Autodesk Fusion 360 part; units mm, degrees
(part 2 of 2)
  spline S41 degree 3 poles (-24.3468, 0.9983) (-24.5744, 0.8236) (-24.8811, 0.6674) (-25.4193, 0.5131) (-25.7453, 0.4822) (-26.274, 0.5385) (-26.5708, 0.63) (-27.014, 0.8762) (-27.2402, 1.07) (-27.3913, 1.2669) (-27.4167, 1.3) (-27.4417, 1.3349) (-27.466, 1.3714) knots -0.320047 -0.320047 -0.320047 -0.320047 -0.233978 -0.233978 -0.152103 -0.152103 -0.074471 -0.074471 0 0 0 0.012509 0.012509 0.012509 0.012509
  spline S42 degree 3 poles (-32.2928, 13.0243) (-32.3014, 13.0672) (-32.3084, 13.1096) (-32.3138, 13.1509) (-32.3462, 13.397) (-32.3233, 13.694) (-32.184, 14.1815) (-32.0388, 14.456) (-31.7048, 14.8697) (-31.4524, 15.0784) (-30.9628, 15.3498) (-30.6354, 15.4563) (-30.351, 15.4937) knots -0.012509 -0.012509 -0.012509 -0.012509 0 0 0 0.074471 0.074471 0.152103 0.152103 0.233978 0.233978 0.320047 0.320047 0.320047 0.320047
  arc A22 (-32.2928, 13.0243) -> (-31.2194, 9.0185) centre (-0.3, 19.45) ccw
  spline S43 degree 3 poles (-28.303, 7.8508) (-28.5681, 7.741) (-28.9049, 7.6694) (-29.4646, 7.6597) (-29.7875, 7.7143) (-30.2836, 7.9055) (-30.5466, 8.0706) (-30.911, 8.4231) (-31.0793, 8.6689) (-31.1743, 8.8983) (-31.1903, 8.9368) (-31.2054, 8.977) (-31.2194, 9.0185) knots -0.320047 -0.320047 -0.320047 -0.320047 -0.233978 -0.233978 -0.152103 -0.152103 -0.074471 -0.074471 0 0 0 0.012509 0.012509 0.012509 0.012509
  spline S44 degree 3 poles (-32.8657, 21.5236) (-32.863, 21.5672) (-32.8587, 21.61) (-32.8533, 21.6513) (-32.8209, 21.8975) (-32.7219, 22.1784) (-32.4612, 22.6132) (-32.2499, 22.8408) (-31.8202, 23.1539) (-31.5224, 23.2902) (-30.9792, 23.4257) (-30.6354, 23.4437) (-30.351, 23.4063) knots -0.012509 -0.012509 -0.012509 -0.012509 0 0 0 0.074471 0.074471 0.152103 0.152103 0.233978 0.233978 0.320047 0.320047 0.320047 0.320047
  arc A23 (-32.8657, 21.5236) -> (-32.8657, 17.3764) centre (-0.3, 19.45) ccw
  spline S45 degree 3 poles (-30.351, 15.4937) (-30.6354, 15.4563) (-30.9792, 15.4743) (-31.5224, 15.6098) (-31.8202, 15.7461) (-32.2499, 16.0592) (-32.4612, 16.2868) (-32.7219, 16.7216) (-32.8209, 17.0025) (-32.8533, 17.2487) (-32.8587, 17.29) (-32.863, 17.3328) (-32.8657, 17.3764) knots -0.320047 -0.320047 -0.320047 -0.320047 -0.233978 -0.233978 -0.152103 -0.152103 -0.074471 -0.074471 0 0 0 0.012509 0.012509 0.012509 0.012509
  spline S46 degree 3 poles (-31.2194, 29.8815) (-31.2054, 29.923) (-31.1903, 29.9632) (-31.1743, 30.0017) (-31.0793, 30.2311) (-30.911, 30.4769) (-30.5466, 30.8294) (-30.2836, 30.9945) (-29.7875, 31.1857) (-29.4646, 31.2403) (-28.9049, 31.2306) (-28.5681, 31.159) (-28.303, 31.0492) knots -0.012509 -0.012509 -0.012509 -0.012509 0 0 0 0.074471 0.074471 0.152103 0.152103 0.233978 0.233978 0.320047 0.320047 0.320047 0.320047
  arc A24 (-31.2194, 29.8815) -> (-32.2928, 25.8757) centre (-0.3, 19.45) ccw
  spline S47 degree 3 poles (-30.351, 23.4063) (-30.6354, 23.4437) (-30.9628, 23.5502) (-31.4524, 23.8216) (-31.7048, 24.0303) (-32.0388, 24.444) (-32.184, 24.7185) (-32.3233, 25.206) (-32.3462, 25.503) (-32.3138, 25.7491) (-32.3084, 25.7904) (-32.3014, 25.8328) (-32.2928, 25.8757) knots -0.320047 -0.320047 -0.320047 -0.320047 -0.233978 -0.233978 -0.152103 -0.152103 -0.074471 -0.074471 0 0 0 0.012509 0.012509 0.012509 0.012509
  line L0 (-22.8918, 33) -> (-17.5918, 33)
  line L1 (-17.5918, 33) -> (-17.5918, 9.5)
  line L2 (-17.5918, 9.5) -> (-22.8918, 9.5)
  line L3 (-22.8918, 9.5) -> (-22.8918, 33)
  circle A25 centre (-0.3, 19.45) radius 4.05
  point P0 (-0.3, 19.45)
  dimension "d1967" = 2.1
  dimension "d2049" = 3
  constraint coincident P0 A0.centre
  measures "d1967" diameter of A0
extrude "Extrude11" add sketch "top_mount" against normal blind 5 contours A25 bodies 5 in component "Cover"
extrude "Extrude6'" cut sketch "top_mount" against normal through all contours A0 bodies 5 in component "Cover"
sketch "Sketch12" plane through (-21.6568, 0, 0) normal (1, 0, 0) x (0, 1, 0) in component "Cover"
  line L0 (-0.1526, -8.2) -> (-0.1526, 19.5)
  line L1 (-2.7, -8.2) -> (-0.1526, -8.2)
  line L2 (-36.2, -8.2) -> (-36.2, 6.4)
  spline S0 degree 3 poles (-19.45, -5.6) (-19.3181, -5.6) (-19.1775, -5.5736) (-18.9188, -5.4665) (-18.8008, -5.3857) (-18.6143, -5.1992) (-18.5335, -5.0812) (-18.4264, -4.8225) (-18.4, -4.6819) (-18.4, -4.4181) (-18.4264, -4.2775) (-18.5335, -4.0188) (-18.6143, -3.9008) (-18.8008, -3.7143) (-18.9188, -3.6335) (-19.1775, -3.5264) (-19.3181, -3.5) (-19.45, -3.5) knots 0.158223 0.158223 0.158223 0.158223 0.197779 0.197779 0.237335 0.237335 0.276891 0.276891 0.316447 0.316447 0.356002 0.356002 0.395558 0.395558 0.435114 0.435114 0.47467 0.47467 0.47467 0.47467 construction
  spline S1 degree 3 poles (-19.45, -3.5) (-19.5819, -3.5) (-19.7225, -3.5264) (-19.9812, -3.6335) (-20.0992, -3.7143) (-20.2857, -3.9008) (-20.3665, -4.0188) (-20.4736, -4.2775) (-20.5, -4.4181) (-20.5, -4.55) (-20.5, -4.6819) (-20.4736, -4.8225) (-20.3665, -5.0812) (-20.2857, -5.1992) (-20.0992, -5.3857) (-19.9812, -5.4665) (-19.7225, -5.5736) (-19.5819, -5.6) (-19.45, -5.6) knots 0.47467 0.47467 0.47467 0.47467 0.514226 0.514226 0.553782 0.553782 0.593337 0.593337 0.632893 0.632893 0.632893 0.672449 0.672449 0.712005 0.712005 0.751561 0.751561 0.791117 0.791117 0.791117 0.791117 construction
  line L3 (-19.45, -5.6) -> (-19.45, -3.5) construction
  circle A0 centre (-19.45, -4.55) radius 1.05
  line L4 (-2.7, -8.2) -> (-5.7, -8.2)
  line L5 (-5.7, -8.2) -> (-5.7, 4.8)
  line L6 (-5.7, 4.8) -> (-2.7, 4.8) construction
  line L7 (-2.7, 4.8) -> (-2.7, -8.2)
  arc A1 (-2.7, 4.8) -> (-5.7, 4.8) centre (-4.2, 4.8) ccw
  line L8 (-36.2, -8.2) -> (-33.2, -8.2)
  line L9 (-36.2, 4.8) -> (-36.2, -8.2)
  arc A2 (-33.2, 4.8) -> (-36.2, 4.8) centre (-34.7, 4.8) ccw
  line L10 (-33.2, -8.2) -> (-33.2, 4.8)
  line L11 (-33.2, 4.8) -> (-36.2, 4.8) construction
  line L12 (-2.7, 6.4) -> (-2.7, -8.2)
  line L13 (-36.2, 6.4) -> (-2.7, 6.4)
  line L14 (-0.1526, 19.5) -> (-38.7474, 19.5)
  line L15 (-38.7474, 19.5) -> (-38.7474, -8.2)
  line L16 (-38.7474, -8.2) -> (-36.2, -8.2)
  dimension "d2042" = 2.1
  dimension "d2043" = 3
  dimension "d2044" = 13
  constraint coincident S0.start S1.end
  constraint coincident S0.end S1.start
  constraint midpoint L3 A0.centre
  constraint horizontal L4
  constraint vertical L5
  constraint horizontal L6
  constraint vertical L7
  constraint coincident L1.start L4.start
  constraint midpoint L6 A1.centre
  constraint symmetric L3 L1.start L2.start
  constraint symmetric L3 L4.end L8.end
  constraint symmetric L3 L5.end A2.start
  constraint symmetric L3 L6.end L9.start
  constraint symmetric L3 A1 A2
  measures "d2042" diameter of A0
  measures "d2043" distance of L1.start L4.end
  measures "d2044" distance of L4.end L5.end
extrude "Extrude10" cut sketch "Sketch12" along normal blind 10 and the other way blind 50 contours L4 L5 L7 A1 L12 | L2 L8 L9 A2 L10 | A0 bodies 5 in component "Cover"
ref_plane "WorkPlane1" through (0.3, -19.45, 1.8046) normal (0, 1, 0) x (1, 0, 0) in component "Hat"
sketch "Sketch1 (2)" plane through (0, -19.45, 0) normal (0, 1, 0) x (1, 0, 0) in component "Hat"
  arc A0 (-32.3317, 6.2002) -> (-32.3317, -21) centre (0.3, -7.3999) ccw
  line L0 (-29.3317, -21) -> (-32.3317, -21)
  arc A1 (-32.3317, -21) -> (-16.0323, -28.2482) centre (-20.3497, -16.0062) ccw
  line L1 (-16.0323, -28.2482) -> (0.267, -22.5)
  line L2 (-16.0323, -28.2482) -> (-16.0323, -21) construction
  line L3 (-32.3317, -21) -> (0.267, -21)
  line L4 (0.267, -21) -> (0.267, -33.2482)
  line L5 (0.267, -33.2482) -> (-2.283, -33.2482)
  line L6 (-2.283, -33.2482) -> (-3.558, -23.8489)
  line L7 (-3.558, -23.8489) -> (-16.0323, -21)
  arc A2 (-2.9205, -28.5486) -> (-8.1816, -22.793) centre (-9.7063, -29.4691) ccw
  line L8 (32.9317, -21) -> (32.8657, -21)
  line L9 (29.3369, 8.2) -> (28.4003, 8.2)
  line L10 (-29.2764, 8.2) -> (-29.3317, 8.2)
  line L11 (-32.3317, -21) -> (32.8657, -21) construction
  dimension "d1949" = 1.5
  dimension "d1956" = 2.55
  dimension "d1991" = 5
  dimension "d1992" = 3.825
  constraint coincident A0.end L0.end
  constraint tangent A0 A1
  constraint tangent A1 L1
  constraint midpoint L2.end L3
  constraint vertical L2
  constraint vertical L4
  constraint coincident L1.end L4
  constraint perpendicular L4 L5
  constraint coincident L1 L6.end
  constraint midpoint L6 A2.start
  constraint tangent L6 A2
  constraint tangent L7 A2
  constraint coincident L7 A2.end
  constraint coincident L8.end L11.end
  constraint midpoint L3.end L11
  measures "d1949" distance of L1.end L3.end
  measures "d1956" distance of L4.end L5.end
  measures "d1991" vertical distance of A1.end L5.end
  measures "d1992" horizontal distance of L3.end L6.end
revolve "Revolve2" add sketch "Sketch1 (2)" angle 360 about axis through (0.267, -19.45, 21) along (0, 0, 1) separate body contours L1 L3 L4 L7 | L1 L7 A2 | L1 L6 A2 | L1 L4 L5 L6 makes body 30 in component "Hat"
revolve "Revolve1'" add sketch "Sketch1 (2)" angle 7.5 about axis through (0.267, -19.45, 21) along (0, 0, -1) second angle 7.5 separate body contours L0 A1 L1 L3 L7 A2 | L1 L3 L4 L7 makes body 31 in component "Hat"
fillet "Fillet1'" radius 2.0665 4 edges at (-10.4771, -20.8645, 26.3218) (-25.4027, -22.8295, 27.8673) (-25.4027, -16.0705, 27.8673) (-10.4771, -18.0355, 26.3218) on bodies 31 in component "Hat"
pattern_circular "C-Pattern1'" count 24 over 360 about axis through (0.267, -19.45, 21) along (0, 0, 1) of bodies 31 makes body 32 at (-19.0466, -24.6251, 21) makes body 33 at (-17.0491, -29.4475, 21) makes body 34 at (-13.8715, -33.5886, 21) makes body 35 at (-9.7304, -36.7661, 21) makes body 36 at (-4.908, -38.7636, 21) makes body 37 at (0.267, -39.4449, 21) makes body 38 at (5.4421, -38.7636, 21) makes body 39 at (10.2645, -36.7661, 21) makes body 40 at (14.4056, -33.5886, 21) makes body 41 at (17.5832, -29.4475, 21) makes body 42 at (19.5807, -24.6251, 21) makes body 43 at (20.262, -19.45, 21) makes body 44 at (19.5807, -14.2749, 21) makes body 45 at (17.5832, -9.4525, 21) makes body 46 at (14.4056, -5.3114, 21) makes body 47 at (10.2645, -2.1339, 21) makes body 48 at (5.4421, -0.1364, 21) makes body 49 at (0.267, 0.5449, 21) makes body 50 at (-4.908, -0.1364, 21) makes body 51 at (-9.7304, -2.1339, 21) makes body 52 at (-13.8715, -5.3114, 21) makes body 53 at (-17.0491, -9.4525, 21) makes body 54 at (-19.0466, -14.2749, 21) in component "Hat"
combine "Combine2" operation add target body 31 tool bodies 44 52 51 37 45 43 54 30 36 41 38 35 32 33 34 39 40 42 48 49 53 47 46 50 in component "Hat"
sketch "Sketch2" plane through (0, 0, 33.2482) normal (0, 0, 1) x (-1, 0, 0) in component "Hat"
  circle A0 centre (-0.267, 19.45) radius 2.55
  circle A1 centre (-0.267, 19.45) radius 1.05
  dimension "d1958" = 2.1
  constraint concentric A0 A1
  measures "d1958" diameter of A1
sketch "profile" plane through (0, 0, 0) normal (1, 0, 0) x (0, 1, 0) in component "Neck"
  line L0 (-40.7, 4.3) -> (-40.7, -19.38)
  line L1 (-40.7, -19.38) -> (2.1, -19.38)
  line L2 (2.1, -19.38) -> (2.1, 4.3)
  line L3 (2.1, 4.3) -> (-2.2, 4.3)
  line L4 (-2.2, 4.3) -> (-2.2, -15.08)
  line L5 (-2.2, -15.08) -> (-36.4, -15.08)
  line L6 (-36.4, -15.08) -> (-36.4, 4.3)
  line L7 (-36.4, 4.3) -> (-40.7, 4.3)
  line L8 (-35.9, -1.2) -> (-35.9, 1.2)
  line L9 (0.6, -2.7) -> (0.6, 2.7)
  line L10 (-3, 2.7) -> (-3, -2.7)
  line L11 (-9.15, -8.2) -> (-28.85, -8.2)
  point P0 (-35.9, 0)
  dimension "d285" = 4.3
  dimension "d286" = 4.3
  dimension "d291" = 0.5
  dimension "d292" = 1.5
  dimension "d293" = 4.3
  dimension "d307" = 6.88
  constraint vertical L0
  constraint perpendicular L0 L1
  constraint perpendicular L1 L2
  constraint perpendicular L2 L3
  constraint perpendicular L3 L4
  constraint perpendicular L4 L5
  constraint perpendicular L5 L6
  constraint perpendicular L6 L7
  constraint equal L3 L7
  constraint collinear L3 L7
  constraint midpoint L8 P0
  measures "d285" distance of L1 L5
  measures "d286" distance of L0.start L6.end
  measures "d291" horizontal distance of L6.end L8.end
  measures "d292" distance of L2 L9
  measures "d293" distance of L7 P0
  measures "d307" distance of L5 L11
extrude "Extrude1''''" add sketch "profile" along normal mid plane 8.6 separate body makes body 55 in component "Neck"
sketch "body_mount" plane through (0, 0, -19.38) normal (0, 0, -1) x (1, 0, 0) in component "Neck"
  line L0 (-4.3, -2.1) -> (4.3, -2.1)
  line L1 (4.3, -2.1) -> (4.3, 40.7)
  line L2 (4.3, 40.7) -> (-4.3, 40.7)
  line L3 (-4.3, 40.7) -> (-4.3, -2.1)
  line L4 (-4.3, 19.3) -> (4.3, 19.3) construction
  circle A0 centre (0, 19.3) radius 0.8
  line L5 (1.3856, 16.9) -> (2.7713, 19.3)
  line L6 (2.7713, 19.3) -> (1.3856, 21.7)
  line L7 (1.3856, 21.7) -> (-1.3856, 21.7)
  line L8 (-1.3856, 21.7) -> (-2.7713, 19.3)
  line L9 (-2.7713, 19.3) -> (-1.3856, 16.9)
  line L10 (-1.3856, 16.9) -> (1.3856, 16.9)
  arc A1 (-4.3, 25.8) -> (-4.3, 12.8) centre (4.3, 19.3) ccw
  line L11 (-4.3, 12.8) -> (-4.3, 25.8)
  point P0 (0, 19.3)
  dimension "d308" = 1.6
  dimension "d309" = 2.4
  dimension "d1880" = 13
  constraint midpoint L3 L4.start
  constraint midpoint L1 L4.end
  constraint midpoint L4 P0
  constraint coincident P0 A0.centre
  constraint horizontal L7
  constraint coincident L3 A1.end
  constraint coincident L3 A1.start
  constraint coincident L4.end A1.centre
  measures "d308" diameter of A0
  measures "d309" distance of P0 L10
  measures "d1880" distance of A1.start A1.end
extrude "Extrude8'" add sketch "body_mount" against normal up to surface (4.3 mm away) contours L3 A1 L11 bodies 55 in component "Neck"
extrude "Extrude2'''" cut sketch "body_mount" against normal up to surface (2.8 mm away) contours A0 | L5 L6 L7 L8 L9 L10 bodies 55 in component "Neck"
extrude "Extrude3''" cut sketch "body_mount" against normal through all contours A0 bodies 55 in component "Neck"
sketch "axis_mount (2)" plane through (0, -40.7, 0) normal (0, -1, 0) x (1, 0, 0) in component "Neck"
  line L0 (-4.3, -19.38) -> (4.3, -19.38)
  line L1 (4.3, -19.38) -> (4.3, 4.3)
  line L2 (4.3, 4.3) -> (-4.3, 4.3)
  line L3 (-4.3, 4.3) -> (-4.3, -19.38)
  circle A0 centre (0, 0) radius 1.05
  line L4 (-2.1, -1.2124) -> (0, -2.4249)
  line L5 (0, -2.4249) -> (2.1, -1.2124)
  line L6 (2.1, -1.2124) -> (2.1, 1.2124)
  line L7 (2.1, 1.2124) -> (0, 2.4249)
  line L8 (0, 2.4249) -> (-2.1, 1.2124)
  line L9 (-2.1, 1.2124) -> (-2.1, -1.2124)
  dimension "d313" = 2.1
  dimension "d314" = 2.1
  constraint coincident A0.centre origin
  constraint vertical L9
  measures "d313" diameter of A0
  measures "d314" distance of A0.centre L9
extrude "Extrude4" cut sketch "axis_mount (2)" along normal blind 2 from surface at -4.3 contours A0 | L4 L5 L6 L7 L8 L9 bodies 55 in component "Neck"
extrude "Extrude5" cut sketch "axis_mount (2)" against normal up to surface (4.3 mm away) contours A0 bodies 55 in component "Neck"
extrude "Extrude2''''" cut sketch "Sketch2" against normal through all contours A1 bodies 31 in component "Hat"
sketch "shaft_mount" plane through (0, 2.1, 0) normal (0, 1, 0) x (-1, 0, 0) in component "Neck"
  line L0 (4.3, 4.3) -> (-4.3, 4.3)
  line L1 (-4.3, 4.3) -> (-4.3, -19.38)
  line L2 (-4.3, -19.38) -> (4.3, -19.38)
  line L3 (4.3, -19.38) -> (4.3, 4.3)
  circle A0 centre (0, 0) radius 0.8
  line L4 (-2.4, -1.3856) -> (0, -2.7713)
  line L5 (0, -2.7713) -> (2.4, -1.3856)
  line L6 (2.4, -1.3856) -> (2.4, 1.3856)
  line L7 (2.4, 1.3856) -> (0, 2.7713)
  line L8 (0, 2.7713) -> (-2.4, 1.3856)
  line L9 (-2.4, 1.3856) -> (-2.4, -1.3856)
  dimension "d320" = 1.6
  dimension "d321" = 2.4
  constraint coincident A0.centre origin
  constraint vertical L6
  measures "d320" diameter of A0
  measures "d321" distance of A0.centre L9
extrude "Extrude6''" cut sketch "shaft_mount" against normal up to surface (2.8 mm away) from surface at -1.5 contours A0 | L4 L5 L6 L7 L8 L9 bodies 55 in component "Neck"
extrude "Extrude7" cut sketch "shaft_mount" against normal up to surface (4.3 mm away) contours A0 bodies 55 in component "Neck"
fillet "Fillet1''" radius 4.3 4 edges at (-4.3, -0.05, 4.3) (4.3, -0.05, 4.3) (-4.3, -38.55, 4.3) (4.3, -38.55, 4.3) on bodies 55 in component "Neck"
fillet "Fillet2" radius 4.3 2 edges at (0, -2.2, -15.08) (0, -36.4, -15.08) on bodies 55 in component "Neck"
fillet "Fillet2" radius 8.6 2 edges at (0, 2.1, -19.38) (0, -40.7, -19.38) on bodies 55 in component "Neck"
component "Servo" placed x (1, 0, 0) y (0, 1, 0) z (0, 0, 1) at (0, 0, 0)
component "OLED" placed x (1, 0, 0) y (0, 1, 0) z (0, 0, 1) at (22.4486, -19.45, 7)
component "Head" placed x (1, 0, 0) y (0, 1, 0) z (0, 0, 1) at (0, 0, 0)
component "Neck" placed x (1, 0, 0) y (0, 1, 0) z (0, 0, 1) at (0, 0, 0)
component "Cover" placed x (1, 0, 0) y (0, 1, 0) z (0, 0, 1) at (-0.1432, 0, 0)
component "Hat" placed x (1, 0, 0) y (0, 1, 0) z (0, 0, 1) at (-0.1102, 0, 0)
equation "servo_body_width = 22.7 mm"
equation "d2 = servo_body_width"
equation "servo_body_height = 17 mm"
equation "servo_mount_width = 4.8 mm"
equation "servo_mount_thickness = 2.4 mm"
equation "d6 = servo_body_height"
equation "d7 = servo_mount_thickness"
equation "d8 = servo_mount_width"
equation "servo_gearbox_height = 4.4 mm"
equation "servo_gearbox_padding = 7.8 mm"
equation "d13 = servo_gearbox_height"
equation "servo_shaft_housing_height = 3.5 mm"
equation "d17 = servo_shaft_position"
equation "servo_shaft_position = 5.8 mm"
equation "servo_shaft_length = 3.3 mm"
equation "d20 = servo_shaft_length"
equation "servo_shaft_radius = 2.4 mm"
equation "servo_body_depth = 12.2 mm"
equation "d23 = servo_body_depth / 2 + servo_clearance"
equation "d25 = ( servo_shaft_radius + servo_clearance ) * 2"
equation "d26 = servo_shaft_length + servo_clearance"
equation "servo_mount_hole_radius = 1.4 mm"
equation "servo_mount_hole_depth_offset = 0 mm"
equation "servo_mount_hole_width_offset = 0.07 mm"
equation "d31 = servo_mount_hole_radius * 2"
equation "d32 = servo_shaft_position"
equation "d33 = servo_mount_width"
equation "d34 = servo_body_depth / 2"
equation "d35 = servo_mount_width / 2 - servo_mount_hole_width_offset"
equation "d36 = servo_body_depth / 2 - servo_mount_hole_depth_offset"
equation "d37 = servo_body_width - servo_shaft_position + servo_mount_width / 2 + servo_mount_hole_width_offset"
equation "servo_clearance = clearance"
equation "d40 = servo_clearance"
equation "min_wall_thickness = 1.5 mm"
equation "oled_width = 36.5 mm"
equation "oled_height = 12.5 mm"
equation "oled_depth = 8.7 mm"
equation "oled_clearance = clearance"
equation "oled_screen_width = 25 mm"
equation "d82 = ( servo_body_height + servo_mount_thickness + servo_gearbox_height ) / 2"
equation "d83 = min(( servo_body_height + servo_mount_thickness + servo_gearbox_height ) - 2 * min_wall_thickness; servo_body_width - 2 * min_wall_thickness)"
equation "d85 = max(0 mm; oled_height - servo_body_depth) + min_wall_thickness"
equation "d87 = -servo_body_depth - 2 * servo_clearance"
equation "d89 = max(screw_thread_diameter + min_wall_thickness; servo_mount_width) + min_wall_thickness"
equation "d90 = max(screw_head_diameter + min_wall_thickness; servo_mount_width) + 0.5 mm"
equation "screw_thread_diameter = 2.1 mm"
equation "screw_head_diameter = 4 mm"
equation "screw_head_height = 2 mm"
equation "d106 = screw_thread_diameter + 0.3 mm"
equation "d115 = servo_shaft_housing_height"
equation "d116 = servo_gearbox_padding"
equation "oled_screen_padding_bottom = 2 mm"
equation "oled_thickness_max = 4.7 mm"
equation "oled_thickness_min = 3.5 mm"
equation "oled_socket_length = 8 mm"
equation "d195 = oled_width"
equation "d196 = oled_thickness_max"
equation "d197 = oled_depth"
equation "d200 = oled_height"
equation "d202 = oled_socket_length"
equation "head_width = d42 + servo_body_height + servo_mount_thickness + servo_gearbox_height + servo_shaft_housing_height + 2 * servo_clearance"
equation "d285 = servo_shaft_length + min_wall_thickness - d291"
equation "d286 = d285"
equation "d292 = min_wall_thickness"
equation "d293 = d285"
equation "d296 = d285"
equation "d301 = d285"
equation "d303 = d285"
equation "d305 = 2 * d285"
equation "d307 = d285 * 1.6"
equation "d309 = servo_shaft_radius"
equation "d310 = -min_wall_thickness"
equation "d313 = screw_thread_diameter"
equation "d321 = servo_shaft_radius"
equation "d322 = -min_wall_thickness"
equation "clearance = 0.3 mm"
equation "d897_1 = 12.00 mm"
equation "d898_1 = 'AI'"
equation "servo_id = 'sg90'"
equation "d1884 = servo_shaft_position"
equation "d1885 = servo_shaft_position"
equation "d1886 = clearance"
equation "d1890 = clearance"
equation "d1891 = clearance"
equation "d1893 = oled_height + oled_clearance * 2"
equation "d1895 = oled_width + 2 * oled_clearance"
equation "d1896 = oled_thickness_max + 2 * oled_clearance"
equation "d1897 = oled_socket_length + 2 * oled_clearance"
equation "d1898 = oled_depth + oled_clearance * 2"
equation "d1899 = min_wall_thickness"
equation "d1914 = oled_clearance"
equation "d1915 = oled_clearance"
equation "d1918 = -clearance"
equation "d1919 = clearance"
equation "d1932 = ( 180 / pumpkin_segments ) * 1 deg"
equation "d1934 = d2054 / 28"
equation "d1935 = ( 180 / pumpkin_segments ) * 1 deg"
equation "d1936 = pumpkin_segments"
equation "d1949 = min_wall_thickness"
equation "d1950 = ( 180 / pumpkin_segments ) * 1 deg"
equation "d1951 = ( 180 / pumpkin_segments ) * 1 deg"
equation "d1953 = d2054 / 28"
equation "d1954 = pumpkin_segments"
equation "d1956 = screw_thread_diameter / 2 + min_wall_thickness"
equation "d1958 = screw_thread_diameter"
equation "d1962 = oled_thickness_min - 2 * oled_clearance"
equation "d1964 = min_wall_thickness"
equation "d1967 = screw_thread_diameter"
equation "d1981 = 2 mm + clearance"
equation "pumpkin_segments = 24"
equation "d1992 = d1956 * 1.5"
equation "d2003 = oled_screen_width - 5 mm"
equation "d2019 = screw_thread_diameter"
equation "d2020 = -min_wall_thickness"
equation "d2027 = screw_thread_diameter"
equation "d2028 = screw_head_diameter"
equation "d2031 = -screw_head_height"
equation "d2035 = min_wall_thickness"
equation "d2042 = screw_thread_diameter"
